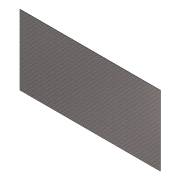
# Autodesk Inventor part: FE-00004-01
Saved by Autodesk Inventor 2012 (Build 160160000, 160)
## iProperties
Created: 2008-05-29
Part Number: FE-00004-01
Document SubType Name: Modeling
Designer: narosenberg
Density: 1 g/cm^3
Description: Panel, Diamond Plate
Mass: 7964.11 g
Surface Area: 33706.4 cm^2
Volume: 7964.11 cm^3
Material: Default
Author: narosenberg
Autodesk Inventor part; units mm, degrees
ref_plane "YZ Plane" through (0, 0, 0) normal (1, 0, 0) x (0, 1, 0)
ref_plane "XZ Plane" through (0, 0, 0) normal (0, 1, 0) x (-1, 0, 0)
sketch "Sketch1" plane through (0, 0, 0) normal (0, 0, 1) x (1, 0, 0)
  line L0 (-35.873, 23.0159) -> (1792.927, 23.0159)
  line L1 (1792.927, 23.0159) -> (1792.927, -891.3841)
  line L2 (1792.927, -891.3841) -> (-35.873, -891.3841)
  line L3 (-35.873, -891.3841) -> (-35.873, 23.0159)
  dimension "d0" = 1828.8
  dimension "d1" = 914.4
  constraints: 8 end point, 2 parallel, 1 horizontal, 1 perpendicular
  measures "d0" distance of L0.start L0.end
  measures "d1" distance of L0.end L1.end
extrude "Extrusion1" add sketch "Sketch1" along normal blind 4.7625
ref_plane "Work Plane1" through (0, 0, 6.0325) normal (0, 0, 1) x (1, 0, 0)
body "Solid1"
